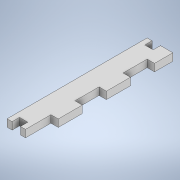
# Autodesk Inventor part: FondV2
Saved by Autodesk Inventor 2020 (Build 240168000, 168)
## iProperties
Created: 2019-11-14
Part Number: FondV2
Material: Générique
Document SubType Name: Modeling
Designer: erwan
Density: 1 g/cm^3
Appearance: Par défaut
Author: erwan
Autodesk Inventor part; units mm, degrees
ref_plane "YZ Plane" through (0, 0, 0) normal (1, 0, 0) x (0, 1, 0)
ref_plane "XZ Plane" through (0, 0, 0) normal (0, 1, 0) x (-1, 0, 0)
ref_plane "XY Plane" through (0, 0, 0) normal (0, 0, 1) x (1, 0, 0)
sketch "Esquisse1" plane through (0, 0, 0) normal (0, 1, 0) x (-1, 0, 0)
  line L0 (0, 0) -> (-15, 0)
  line L1 (-55, -419) -> (-40, -419)
  line L2 (0, -419) -> (0, 0)
  line L3 (-40, -419) -> (-40, -397)
  line L4 (-40, -397) -> (-15, -397)
  line L5 (-15, -397) -> (-15, -419)
  line L6 (-15, -419) -> (0, -419)
  line L7 (-40, 0) -> (-40, -22)
  line L8 (-40, -22) -> (-15, -22)
  line L9 (-15, -22) -> (-15, 0)
  line L10 (-40, 0) -> (-55, 0)
  line L11 (-55, 0) -> (-55, -76)
  line L12 (-55, -76) -> (-77, -76)
  line L13 (-77, -76) -> (-77, -148)
  line L14 (-77, -148) -> (-55, -148)
  line L15 (-55, -148) -> (-55, -220)
  line L16 (-55, -220) -> (-77, -220)
  line L17 (-77, -220) -> (-77, -292)
  line L18 (-77, -292) -> (-55, -292)
  line L19 (-55, -292) -> (-55, -364)
  line L20 (-55, -364) -> (-77, -364)
  line L21 (-77, -364) -> (-77, -419)
  line L22 (-77, -419) -> (-55, -419)
  dimension "d0" = 419
  dimension "d2" = 22
  dimension "d3" = 25
  dimension "d4" = 15
  dimension "d6" = 22
  dimension "d7" = 25
  dimension "d8" = 15
  dimension "d12" = 76
  dimension "d13" = 22
  dimension "d14" = 72
  dimension "d15" = 72
  dimension "d16" = 72
  dimension "d17" = 72
  constraints: 46 end point, 7 perpendicular, 6 parallel, 6 point on line, 2 horizontal, 2 vertical
  measures "d0" distance between parallel lines of L0 L1
  measures "d2" distance between parallel lines of L4 L1
  measures "d3" distance between parallel lines of L3 L5
  measures "d4" distance between parallel lines of L5 L2
  measures "d6" distance between parallel lines of L0 L8
  measures "d7" distance between parallel lines of L7 L9
  measures "d8" distance between parallel lines of L2 L9
  measures "d12" distance of L10.end L11.end
  measures "d13" distance of L11.end L12.end
  measures "d14" distance of L12.end L13.end
  measures "d15" distance of L14.end L15.end
  measures "d16" distance of L16.end L17.end
  measures "d17" distance of L18.end L19.end
extrude "Extrusion1" add sketch "Esquisse1" along normal blind 22
